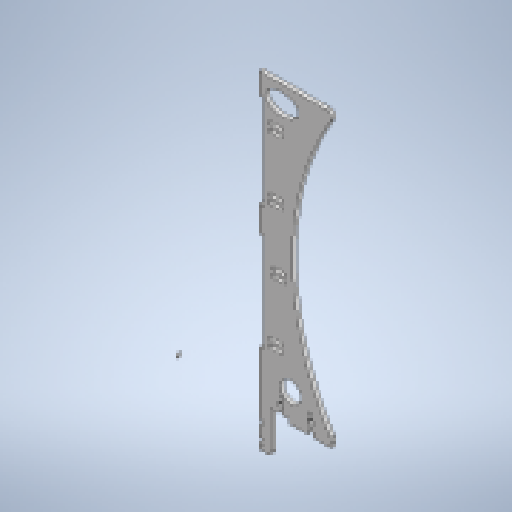
# Autodesk Inventor part: ребро
Saved by Autodesk Inventor 2023.1 (Build 271208000, 208)
## iProperties
Created: 2025-01-17
Part Number: ребро
Material: Типовые
Document SubType Name: Modeling
Designer: Коноваленко
Density: 1 g/cm^3
Appearance: По умолчанию
Author: Коноваленко
Autodesk Inventor part; units mm, degrees
ref_plane "YZ Plane" through (0, 0, 0) normal (1, 0, 0) x (0, 1, 0)
ref_plane "XZ Plane" through (0, 0, 0) normal (0, 1, 0) x (-1, 0, 0)
ref_plane "XY Plane" through (0, 0, 0) normal (0, 0, 1) x (1, 0, 0)
sketch "Эскиз1" plane through (0, 0, 0) normal (0, 0, 1) x (1, 0, 0)
  line L0 (81.8324, 0) -> (81.8324, -4) construction
  line L1 (72.759, -4) -> (11.9953, -4)
  line L2 (11.9953, -4) -> (11.9953, 0) construction
  line L3 (11.9953, 0) -> (81.8324, 0) construction
  line L4 (-75.5314, 0) -> (7.9958, 0) construction
  line L5 (7.9958, 0) -> (7.9958, -4) construction
  line L6 (7.9958, -4) -> (-66.4579, -4)
  line L7 (-75.5314, -4) -> (-75.5314, 0) construction
  line L8 (7.9953, 276) -> (11.9953, 276) construction
  line L9 (-75.5314, 0) -> (81.8324, 0)
  line L10 (72.759, 276) -> (-66.4579, 276)
  arc A0 (-70.7311, 3.5962) -> (-70.7311, 268.4038) centre (-288.6628, 136) ccw
  line L11 (3.1505, 276) -> (3.1505, 0) construction
  arc A1 (77.0322, 268.4038) -> (77.0322, 3.5962) centre (294.9639, 136) ccw
  arc A2 (-66.4579, 276) -> (-70.7311, 268.4038) centre (-66.4579, 271) ccw
  arc A3 (77.0322, 268.4038) -> (72.759, 276) centre (72.759, 271) ccw
  arc A4 (-70.7311, 3.5962) -> (-66.4579, -4) centre (-66.4579, 1) ccw
  arc A5 (72.759, -4) -> (77.0322, 3.5962) centre (72.759, 1) ccw
  point P0 (81.8324, 276)
  point P1 (-75.5314, 276)
  point P2 (-71.3569, 0)
  point P3 (77.658, 0)
  dimension "d0" = 255
  dimension "d1" = 5
  constraints: 24 end point, 16 point on circle, 8 tangent, 6 centre point, 4 point on line, 3 equal radius, 2 midpoint, 1 horizontal, 1 parallel, 1 symmetric about line, 1 other
  measures "d0" radius of A0
  measures "d1" radius of A2
extrude "Выдавливание1" add sketch "Эскиз1" along normal blind 4
sketch "Эскиз2" plane through (0, 0, 4) normal (0, 0, 1) x (1, 0, 0)
  line L0 (-29.8867, 53.1563) -> (-17.8867, 53.1563)
  line L1 (42.1133, 53.1563) -> (42.1133, 54.9927) construction
  line L2 (-29.8867, 50.1563) -> (-29.8867, 53.1563)
  line L3 (6.1133, 50.1563) -> (6.1133, 53.1563)
  line L4 (6.1133, 50.1563) -> (6.1133, 53.1563) construction
  line L5 (-17.8867, 50.1563) -> (-17.8867, 53.1563)
  line L6 (-5.8867, 50.1563) -> (-5.8867, 53.1563)
  line L7 (18.1133, 50.1563) -> (18.1133, 53.1563)
  line L8 (30.1133, 50.1563) -> (30.1133, 53.1563)
  line L9 (-17.8867, 50.1563) -> (-29.8867, 50.1563)
  line L10 (-17.8867, 53.1563) -> (-5.8867, 53.1563) construction
  line L11 (-5.8867, 53.1563) -> (6.1133, 53.1563)
  line L12 (-5.8867, 50.1563) -> (-17.8867, 50.1563) construction
  line L13 (6.1133, 53.1563) -> (18.1133, 53.1563) construction
  line L14 (18.1133, 50.1563) -> (6.1133, 50.1563) construction
  line L15 (18.1133, 53.1563) -> (30.1133, 53.1563)
  line L16 (30.1133, 53.1563) -> (42.1133, 53.1563) construction
  line L17 (30.1133, 50.1563) -> (18.1133, 50.1563)
  line L18 (6.1133, 50.1563) -> (-5.8867, 50.1563)
  line L19 (6.1133, 6.0367) -> (6.1133, 56.3563) construction
  line L20 (-29.8867, 59.3563) -> (-17.8867, 59.3563)
  line L21 (42.1133, 59.3563) -> (42.1133, 56.3563) construction
  line L22 (42.1133, 56.3563) -> (30.1133, 56.3563) construction
  line L23 (-29.8867, 56.3563) -> (-29.8867, 59.3563)
  line L24 (6.1133, 56.3563) -> (6.1133, 59.3563)
  line L25 (6.1133, 56.3563) -> (6.1133, 59.3563) construction
  line L26 (-17.8867, 56.3563) -> (-17.8867, 59.3563)
  line L27 (-5.8867, 56.3563) -> (-5.8867, 59.3563)
  line L28 (18.1133, 56.3563) -> (18.1133, 59.3563)
  line L29 (30.1133, 56.3563) -> (30.1133, 59.3563)
  line L30 (-17.8867, 56.3563) -> (-29.8867, 56.3563)
  line L31 (-17.8867, 59.3563) -> (-5.8867, 59.3563) construction
  line L32 (-5.8867, 59.3563) -> (6.1133, 59.3563)
  line L33 (-5.8867, 56.3563) -> (-17.8867, 56.3563) construction
  line L34 (6.1133, 59.3563) -> (18.1133, 59.3563) construction
  line L35 (18.1133, 56.3563) -> (6.1133, 56.3563) construction
  line L36 (18.1133, 59.3563) -> (30.1133, 59.3563)
  line L37 (30.1133, 59.3563) -> (42.1133, 59.3563) construction
  line L38 (30.1133, 56.3563) -> (18.1133, 56.3563)
  line L39 (6.1133, 56.3563) -> (-5.8867, 56.3563)
  line L40 (6.1133, -16.2034) -> (6.1133, 259.7966) construction
  line L41 (72.759, 276) -> (-66.4579, 276) projected
  line L42 (9.151, 110.1563) -> (9.151, 113.1563)
  line L43 (9.151, 110.1563) -> (9.151, 113.1563) construction
  line L44 (-2.8491, 113.1563) -> (9.151, 113.1563)
  line L45 (9.151, 110.1563) -> (-2.8491, 110.1563)
  line L46 (-2.8491, 110.1563) -> (-2.8491, 113.1563)
  line L47 (-14.8491, 110.1563) -> (-14.8491, 113.1563)
  line L48 (-14.8491, 113.1563) -> (-2.8491, 113.1563) construction
  line L49 (-2.8491, 110.1563) -> (-14.8491, 110.1563) construction
  line L50 (9.151, 55.0001) -> (9.151, 110.1563) construction
  line L51 (21.151, 110.1563) -> (9.151, 110.1563) construction
  line L52 (9.151, 113.1563) -> (21.151, 113.1563) construction
  line L53 (21.151, 110.1563) -> (21.151, 113.1563)
  line L54 (33.151, 110.1563) -> (21.151, 110.1563)
  line L55 (21.151, 113.1563) -> (33.151, 113.1563)
  line L56 (33.151, 110.1563) -> (33.151, 113.1563)
  line L57 (45.1508, 113.1563) -> (45.1508, 110.1563) construction
  line L58 (33.151, 113.1563) -> (45.1508, 113.1563) construction
  line L59 (-26.8491, 113.1563) -> (-14.8491, 113.1563)
  line L60 (-26.8491, 110.1563) -> (-26.8491, 113.1563)
  line L61 (-14.8491, 110.1563) -> (-26.8491, 110.1563)
  line L62 (-14.7363, 116.3563) -> (-14.7363, 119.3563)
  line L63 (-26.7363, 119.3563) -> (-14.7363, 119.3563)
  line L64 (-14.7363, 116.3563) -> (-26.7363, 116.3563)
  line L65 (21.2639, 116.3563) -> (21.2639, 119.3563)
  line L66 (21.2639, 119.3563) -> (33.2639, 119.3563)
  line L67 (33.2639, 116.3563) -> (33.2639, 119.3563)
  line L68 (33.2639, 116.3563) -> (21.2639, 116.3563)
  line L69 (45.2637, 119.3563) -> (45.2637, 116.3563) construction
  line L70 (21.2639, 116.3563) -> (9.2639, 116.3563) construction
  line L71 (9.2639, 119.3563) -> (21.2639, 119.3563) construction
  line L72 (9.2639, 116.3563) -> (9.2639, 119.3563)
  line L73 (9.2639, 116.3563) -> (9.2639, 119.3563) construction
  line L74 (-26.7363, 116.3563) -> (-26.7363, 119.3563)
  line L75 (33.2639, 119.3563) -> (45.2637, 119.3563) construction
  line L76 (-14.7363, 119.3563) -> (-2.7363, 119.3563) construction
  line L77 (-2.7363, 116.3563) -> (-2.7363, 119.3563)
  line L78 (-2.7363, 119.3563) -> (9.2639, 119.3563)
  line L79 (9.2639, 116.3563) -> (-2.7363, 116.3563)
  line L80 (-2.7363, 116.3563) -> (-14.7363, 116.3563) construction
  line L81 (45.2637, 116.3563) -> (33.2639, 116.3563) construction
  line L82 (6.1133, 170.1563) -> (6.1133, 173.1563)
  line L83 (6.1133, 170.1563) -> (6.1133, 173.1563) construction
  line L84 (-5.8867, 173.1563) -> (6.1133, 173.1563)
  line L85 (6.1133, 170.1563) -> (-5.8867, 170.1563)
  line L86 (-5.8867, 170.1563) -> (-5.8867, 173.1563)
  line L87 (-17.8867, 170.1563) -> (-17.8867, 173.1563)
  line L88 (-17.8867, 173.1563) -> (-5.8867, 173.1563) construction
  line L89 (-5.8867, 170.1563) -> (-17.8867, 170.1563) construction
  line L90 (18.1133, 170.1563) -> (6.1133, 170.1563) construction
  line L91 (6.1133, 173.1563) -> (18.1133, 173.1563) construction
  line L92 (18.1133, 170.1563) -> (18.1133, 173.1563)
  line L93 (30.1133, 170.1563) -> (18.1133, 170.1563)
  line L94 (18.1133, 173.1563) -> (30.1133, 173.1563)
  line L95 (30.1133, 170.1563) -> (30.1133, 173.1563)
  line L96 (42.1133, 170.1563) -> (30.1133, 170.1563) construction
  line L97 (42.1133, 173.1563) -> (42.1133, 170.1563) construction
  line L98 (30.1133, 173.1563) -> (42.1133, 173.1563) construction
  line L99 (-29.8867, 173.1563) -> (-17.8867, 173.1563)
  line L100 (-29.8867, 170.1563) -> (-29.8867, 173.1563)
  line L101 (-17.8867, 170.1563) -> (-29.8867, 170.1563)
  line L102 (6.1133, 179.3563) -> (18.1133, 179.3563) construction
  line L103 (18.1133, 176.3563) -> (6.1133, 176.3563) construction
  line L104 (18.1133, 176.3563) -> (18.1133, 179.3563)
  line L105 (30.1133, 176.3563) -> (18.1133, 176.3563)
  line L106 (18.1133, 179.3563) -> (30.1133, 179.3563)
  line L107 (-29.8867, 179.3563) -> (-17.8867, 179.3563)
  line L108 (-17.8867, 176.3563) -> (-29.8867, 176.3563)
  line L109 (-29.8867, 176.3563) -> (-29.8867, 179.3563)
  line L110 (-17.8867, 176.3563) -> (-17.8867, 179.3563)
  line L111 (30.1133, 176.3563) -> (30.1133, 179.3563)
  line L112 (42.1133, 176.3563) -> (30.1133, 176.3563) construction
  line L113 (42.1133, 179.3563) -> (42.1133, 176.3563) construction
  line L114 (30.1133, 179.3563) -> (42.1133, 179.3563) construction
  line L115 (-5.8867, 176.3563) -> (-17.8867, 176.3563) construction
  line L116 (-17.8867, 179.3563) -> (-5.8867, 179.3563) construction
  line L117 (-5.8867, 176.3563) -> (-5.8867, 179.3563)
  line L118 (6.1133, 176.3563) -> (-5.8867, 176.3563)
  line L119 (-5.8867, 179.3563) -> (6.1133, 179.3563)
  line L120 (6.1133, 176.3563) -> (6.1133, 179.3563)
  line L121 (6.1133, 176.3563) -> (6.1133, 179.3563) construction
  line L122 (6.1133, 233.1563) -> (18.1133, 233.1563) construction
  line L123 (18.1133, 230.1563) -> (6.1133, 230.1563) construction
  line L124 (18.1133, 230.1563) -> (18.1133, 233.1563)
  line L125 (30.1133, 230.1563) -> (18.1133, 230.1563)
  line L126 (18.1133, 233.1563) -> (30.1133, 233.1563)
  line L127 (-29.8867, 233.1563) -> (-17.8867, 233.1563)
  line L128 (-17.8867, 230.1563) -> (-29.8867, 230.1563)
  line L129 (-29.8867, 230.1563) -> (-29.8867, 233.1563)
  line L130 (-17.8867, 230.1563) -> (-17.8867, 233.1563)
  line L131 (30.1133, 230.1563) -> (30.1133, 233.1563)
  line L132 (42.1133, 230.1563) -> (30.1133, 230.1563) construction
  line L133 (42.1133, 233.1563) -> (42.1133, 230.1563) construction
  line L134 (30.1133, 233.1563) -> (42.1133, 233.1563) construction
  line L135 (-5.8867, 230.1563) -> (-17.8867, 230.1563) construction
  line L136 (-17.8867, 233.1563) -> (-5.8867, 233.1563) construction
  line L137 (-5.8867, 230.1563) -> (-5.8867, 233.1563)
  line L138 (6.1133, 230.1563) -> (-5.8867, 230.1563)
  line L139 (-5.8867, 233.1563) -> (6.1133, 233.1563)
  line L140 (6.1133, 230.1563) -> (6.1133, 233.1563)
  line L141 (6.1133, 230.1563) -> (6.1133, 233.1563) construction
  line L142 (18.1133, 236.3563) -> (18.1133, 239.3563)
  line L143 (30.1133, 236.3563) -> (18.1133, 236.3563)
  line L144 (18.1133, 239.3563) -> (30.1133, 239.3563)
  line L145 (30.1133, 236.3563) -> (30.1133, 239.3563)
  line L146 (42.1133, 236.3563) -> (30.1133, 236.3563) construction
  line L147 (30.1133, 239.3563) -> (42.1133, 239.3563) construction
  line L148 (42.1133, 239.3563) -> (42.1133, 236.3563) construction
  line L149 (18.1133, 236.3563) -> (6.1133, 236.3563) construction
  line L150 (6.1133, 239.3563) -> (18.1133, 239.3563) construction
  line L151 (6.1133, 236.3563) -> (6.1133, 239.3563)
  line L152 (6.1133, 236.3563) -> (6.1133, 239.3563) construction
  line L153 (6.1133, 236.3563) -> (-5.8867, 236.3563)
  line L154 (-5.8867, 239.3563) -> (6.1133, 239.3563)
  line L155 (-5.8867, 236.3563) -> (-5.8867, 239.3563)
  line L156 (-5.8867, 236.3563) -> (-17.8867, 236.3563) construction
  line L157 (-17.8867, 239.3563) -> (-5.8867, 239.3563) construction
  line L158 (-17.8867, 236.3563) -> (-17.8867, 239.3563)
  line L159 (-29.8867, 239.3563) -> (-17.8867, 239.3563)
  line L160 (-29.8867, 236.3563) -> (-29.8867, 239.3563)
  line L161 (-17.8867, 236.3563) -> (-29.8867, 236.3563)
  arc A0 (-70.7311, 3.5962) -> (-70.7311, 268.4038) centre (-288.6628, 136) ccw construction
  arc A1 (77.0322, 268.4038) -> (77.0322, 3.5962) centre (294.9639, 136) ccw construction
  line L162 (11.994, 110.1563) -> (7.994, 110.1563)
  line L163 (11.9939, 170.1563) -> (7.9939, 170.1563)
  line L164 (11.9939, 230.1563) -> (7.9939, 230.1563)
  point P0 (0, 0)
  point P1 (-29.8867, 51.6563)
  point P2 (-17.8867, 51.6563)
  point P3 (-5.8867, 51.6563)
  point P4 (6.1133, 51.6563)
  point P5 (18.1133, 51.6563)
  point P6 (30.1133, 51.6563)
  point P7 (6.1133, 57.8563)
  point P8 (-29.8867, 57.8563)
  point P9 (-17.8867, 57.8563)
  point P10 (-5.8867, 57.8563)
  point P11 (6.1133, 57.8563)
  point P12 (18.1133, 57.8563)
  point P13 (30.1133, 57.8563)
  point P14 (6.1133, 117.4846)
  point P15 (9.2638, 118.9846)
  point P16 (9.151, 111.6563)
  point P17 (-2.8491, 111.6563)
  point P18 (21.151, 111.6563)
  point P19 (33.151, 111.6563)
  point P20 (-14.8491, 111.6563)
  point P21 (-26.8491, 111.6563)
  point P22 (6.1133, 123.6846)
  point P23 (6.1133, 123.6846)
  point P24 (21.2639, 117.8563)
  point P25 (33.2639, 117.8563)
  point P26 (9.2639, 117.8563)
  point P27 (-26.7363, 117.8563)
  point P28 (-2.7363, 117.8563)
  point P29 (-14.7363, 117.8563)
  point P30 (9.2638, 125.1846)
  point P31 (3.2638, 119.3563)
  point P32 (30.1133, 171.6563)
  point P33 (-17.8867, 171.6563)
  point P34 (-29.8867, 171.6563)
  point P35 (6.1133, 177.1846)
  point P36 (-17.8867, 177.8563)
  point P37 (-29.8867, 177.8563)
  point P38 (30.1133, 177.8563)
  point P39 (6.1133, 177.8563)
  point P40 (6.1133, 225.9846)
  point P41 (6.1133, 225.9846)
  point P42 (18.1133, 231.6563)
  point P43 (-17.8867, 231.6563)
  point P44 (-29.8867, 231.6563)
  point P45 (30.1133, 231.6563)
  point P46 (-5.8867, 231.6563)
  point P47 (18.1133, 237.8563)
  point P48 (30.1133, 237.8563)
  point P49 (-5.8867, 237.8563)
  point P50 (-17.8867, 237.8563)
  point P51 (-29.8867, 237.8563)
  point P52 (6.1133, 232.1846)
  point P53 (6.1133, 225.1563)
  point P54 (0.1133, 179.3563)
  point P55 (9.994, 50.1563)
  point P56 (9.994, 110.1563)
  point P57 (9.9939, 170.1563)
  point P58 (9.9939, 230.1563)
  dimension "d18" = 12
  dimension "d19" = 12
  dimension "d20" = 12
  dimension "d21" = 12
  dimension "d22" = 4.7
  dimension "d23" = 72
  dimension "d25" = 12
  dimension "d26" = 12
  dimension "d27" = 12
  dimension "d28" = 12
  dimension "d39" = 12
  dimension "d40" = 12
  dimension "d41" = 12
  dimension "d42" = 12
  dimension "d44" = 72
  dimension "d46" = 12
  dimension "d47" = 12
  dimension "d48" = 12
  dimension "d49" = 12
  dimension "d54" = 12
  dimension "d59" = 72
  dimension "d60" = 3
  dimension "d61" = 12
  dimension "d66" = 72
  dimension "d68" = 12
  dimension "d69" = 12
  dimension "d71" = 12
  dimension "d74" = 3
  dimension "d75" = 12
  dimension "d76" = 12
  dimension "d78" = 12
  dimension "d79" = 45.8
  dimension "d97" = 3.2
  dimension "d98" = 3
  dimension "d99" = 3.2
  dimension "d100" = 3
  dimension "d101" = 3.2
  dimension "d102" = 3.2
  constraints: 328 end point, 284 parallel, 238 perpendicular, 91 point on line, 48 horizontal, 46 midpoint, 11 vertical, 8 equal length
  measures "d18" distance of point (-29.887, 51.656) point (-17.887, 51.656)
  measures "d19" distance of point (-5.887, 51.656) point (-17.887, 51.656)
  measures "d20" distance of point (6.113, 51.656) point (18.113, 51.656)
  measures "d21" distance of point (30.113, 51.656) point (18.113, 51.656)
  measures "d22" distance from line of point (6.113, 57.856) L11
  measures "d23" distance of L22.start L23.start
  measures "d25" distance of point (-29.887, 57.856) point (-17.887, 57.856)
  measures "d26" distance of point (-5.887, 57.856) point (-17.887, 57.856)
  measures "d27" distance of point (6.113, 57.856) point (18.113, 57.856)
  measures "d28" distance of point (30.113, 57.856) point (18.113, 57.856)
  measures "d39" distance of point (-26.849, 111.656) point (-14.849, 111.656)
  measures "d40" distance of point (-2.849, 111.656) point (-14.849, 111.656)
  measures "d41" distance of point (9.151, 111.656) point (21.151, 111.656)
  measures "d42" distance of point (33.151, 111.656) point (21.151, 111.656)
  measures "d44" distance of L81.start L64.end
  measures "d46" distance of point (-26.736, 117.856) point (-14.736, 117.856)
  measures "d47" distance of point (-2.736, 117.856) point (-14.736, 117.856)
  measures "d48" distance of point (9.264, 117.856) point (21.264, 117.856)
  measures "d49" distance of point (33.264, 117.856) point (21.264, 117.856)
  measures "d54" distance of point (-29.887, 171.656) point (-17.887, 171.656)
  measures "d59" distance of L112.start L109.start
  measures "d60" distance of L114.end L112.start
  measures "d61" distance of point (-29.887, 177.856) point (-17.887, 177.856)
  measures "d66" distance of L132.start L128.end
  measures "d68" distance of point (-29.887, 231.656) point (-17.887, 231.656)
  measures "d69" distance of point (-5.887, 231.656) point (-17.887, 231.656)
  measures "d71" distance of point (30.113, 231.656) point (18.113, 231.656)
  measures "d74" distance of L147.end L146.start
  measures "d75" distance of point (-29.887, 237.856) point (-17.887, 237.856)
  measures "d76" distance of point (-5.887, 237.856) point (-17.887, 237.856)
  measures "d78" distance of point (30.113, 237.856) point (18.113, 237.856)
  measures "d79" vertical distance of point (6.113, 225.156) point (0.113, 179.356)
  measures "d97" distance of L0.start L23.start
  measures "d98" distance of L8.start L8.end
  measures "d99" distance between parallel lines of L55 L68
  measures "d100" distance of L61.end L59.start
  measures "d101" distance between parallel lines of L94 L105
  measures "d102" distance between parallel lines of L126 L143
extrude "Выдавливание2" cut sketch "Эскиз2" against normal blind 10
sketch "Эскиз3" plane through (0, 0, 0) normal (0, 0, -1) x (-1, 0, 0)
  line L0 (29.8867, 239.3563) -> (29.8867, 236.3563)
  line L1 (5.8867, 236.3563) -> (5.8867, 239.3563) construction
  line L2 (29.8867, 239.3563) -> (17.8867, 239.3563) construction
  line L3 (5.8867, 239.3563) -> (17.8867, 239.3563) construction
  line L4 (17.8867, 239.3563) -> (17.8867, 287.0573) construction
  line L5 (-72.759, 276) -> (66.4579, 276) construction
  line L6 (-72.759, 276) -> (66.4579, 276) projected
  line L7 (-3.1505, 276) -> (-3.1505, 0) construction
  ellipse E0 centre (14.7363, 209.3563) end of major axis (14.7363, 194.3563) minor radius 10
  ellipse E1 centre (14.7363, 149.3563) end of major axis (14.7363, 134.3563) minor radius 10
  line L8 (26.9628, 119.3563) -> (14.9628, 119.3563) construction
  line L9 (14.9628, 119.3563) -> (26.9628, 119.3563)
  ellipse E2 centre (-30.1133, 259.231) end of major axis (-46.1133, 259.231) minor radius 10
  line L10 (-30.1133, 236.3563) -> (-30.1133, 239.3563) projected
  line L11 (-18.1133, 239.3563) -> (-30.1133, 239.3563) projected
  line L12 (-30.1133, 239.3563) -> (-30.1133, 283.7222) construction
  line L13 (26.7363, 119.3563) -> (14.7363, 119.3563) projected
  line L14 (14.7363, 119.3563) -> (14.7363, 279.8353) construction
  line L15 (14.7363, 119.3563) -> (175.2153, 119.3563) construction
  line L16 (14.7363, 119.3563) -> (14.7363, -15.3407) construction
  ellipse E3 centre (14.7363, 87.8563) end of major axis (14.7363, 72.8563) minor radius 10
  ellipse E4 centre (14.7363, 29.3563) end of major axis (14.7363, 14.3563) minor radius 10
  line L17 (14.7363, 116.3563) -> (14.7363, 119.3563) projected
  point P0 (0, 0)
  point P1 (-33.2639, 119.3563)
  point P2 (-21.2639, 119.3563)
  point P3 (17.8867, 179.3563)
  point P4 (17.8867, 59.3563)
  point P5 (14.7363, 117.8563)
  dimension "d92" = 16
  dimension "d90" = 160.479
  dimension "d91" = 90
  dimension "d93" = 30
  dimension "d94" = 30
  dimension "d95" = 30
  dimension "d96" = 30
  constraints: 20 end point, 5 point on line, 4 centre point, 3 perpendicular, 3 vertical, 2 horizontal, 2 midpoint, 2 symmetric about line, 2 other
  measures "d90" distance of L13.end L14.end
  measures "d91" angle of L15 L14
  measures "d93" vertical distance of L2.end E0.centre
  measures "d94" vertical distance of E1.centre point (17.887, 179.356)
  measures "d95" distance of E3.centre point (14.736, 117.856)
  measures "d96" vertical distance of E4.centre point (17.887, 59.356)
extrude "Выдавливание3" cut sketch "Эскиз3" against normal blind 10
sketch "Эскиз4" plane through (-71.3569, 0, 0) normal (0, -1, 0) x (1, 0, 0)
  line L0 (91.3569, 4) -> (51.3569, 4)
  line L1 (51.3569, 4) -> (51.3569, 0)
  line L2 (51.3569, 0) -> (91.3569, 0)
  line L3 (91.3569, 0) -> (91.3569, 4)
  line L4 (72.8558, 3.5003) -> (72.8557, 3.5003) projected
  point P0 (71.3569, 0)
  point P1 (0, 4)
  point P2 (149.0149, 4)
  dimension "d103" = 40
  dimension "d104" = 4
  constraints: 8 end point, 2 parallel, 1 horizontal, 1 midpoint, 1 perpendicular
  measures "d103" distance of L1.end L2.end
  measures "d104" distance of L0.end L1.end
extrude "Выдавливание4" add sketch "Эскиз4" along normal blind 20
sketch "Эскиз5" plane through (0, 0, 0) normal (0, 0, -1) x (-1, 0, 0)
  line L0 (0, -20) -> (-20, -20)
  line L1 (-20, -20) -> (-20, -40)
  line L2 (-20, -40) -> (0, -40)
  line L3 (0, -40) -> (0, -20)
  line L4 (20, -20) -> (-20, -20) projected
  point P0 (0, 0)
  point P1 (17, -20)
  point P2 (-17, -20)
  point P3 (0, -20)
  dimension "d108" = 20
  dimension "d109" = 20
  constraints: 8 end point, 2 parallel, 1 horizontal, 1 midpoint, 1 perpendicular
  measures "d108" distance of L2.end L1.end
  measures "d109" distance of L0.end L1.end
extrude "Выдавливание5" add sketch "Эскиз5" against normal blind 4
fillet "Сопряжение2" radius 3 3 edges at (20, -40, 2) (0, -40, 2) (0, -20, 2)
fillet "Сопряжение3" radius 3 1 edges at (-20, -20, 2)
sketch "Эскиз6" plane through (0, 0, 0) normal (0, 0, -1) x (-1, 0, 0)
  line L0 (0, -37) -> (0, -23) projected
  line L1 (-20, 0) -> (-20, -37) projected
  line L2 (0, -23) -> (0, -37) projected
  circle A0 centre (-10, -32) radius 2.55
  circle A1 centre (-10, -17) radius 2.55
  line L3 (-10, -17) -> (-10, -32) construction
  line L4 (-17, -40) -> (-3, -40) projected
  line L5 (-10, -32) -> (-20, -32) construction
  line L6 (-10, -32) -> (0, -32) construction
  point P0 (0, 0)
  point P1 (-10, -40)
  dimension "d121" = 5.1
  dimension "d122" = 5.1
  dimension "d123" = 8
  dimension "d124" = 15
  constraints: 6 end point, 3 point on line, 2 centre point, 1 collinear, 1 midpoint, 1 parallel, 1 perpendicular
  measures "d121" diameter of A1
  measures "d122" diameter of A0
  measures "d123" distance of point (-10, -40) L3.end
  measures "d124" distance of L3.start L3.end
extrude "Выдавливание6" cut sketch "Эскиз6" against normal blind 4
sketch "Эскиз7" plane through (0, 0, 0) normal (0, 0, -1) x (-1, 0, 0)
  circle A0 centre (-38.6107, 23.1063) radius 10
  point P0 (0, 0)
  dimension "d125" = 20
  constraints: 1 centre point
  measures "d125" diameter of A0
extrude "Выдавливание7" cut sketch "Эскиз7" against normal blind 4
sketch "Эскиз8" plane through (77.658, 0, 0) normal (0, -1, 0) x (1, 0, 0)
  line L0 (-57.658, 4) -> (0, 4) construction
  line L1 (-57.658, 0) -> (0, 0) construction
  line L2 (0, 4) -> (-17.5, 4)
  line L3 (-17.5, 4) -> (-17.5, 0)
  line L4 (-17.5, 0) -> (0, 0)
  line L5 (0, 0) -> (0, 4)
  line L6 (-22.5, 4) -> (-40, 4)
  line L7 (-40, 4) -> (-40, 0)
  line L8 (-40, 0) -> (-22.5, 0)
  line L9 (-22.5, 0) -> (-22.5, 4)
  line L10 (-148.3891, 0) -> (-149.1159, 0) projected
  line L11 (-149.0149, 4) -> (-97.658, 4) projected
  line L12 (-149.1159, 0) -> (-131.6159, 0)
  line L13 (-131.6159, 0) -> (-131.6159, 4)
  line L14 (-131.6159, 4) -> (-149.1159, 4)
  line L15 (-149.1159, 4) -> (-149.1159, 0)
  line L16 (-149.0149, 0) -> (-97.658, 0) projected
  line L17 (-126.6159, 0) -> (-109.1159, 0)
  line L18 (-109.1159, 0) -> (-109.1159, 4)
  line L19 (-109.1159, 4) -> (-126.6159, 4)
  line L20 (-126.6159, 4) -> (-126.6159, 0)
  point P0 (-77.658, 0)
  point P1 (-17.5, 4)
  point P2 (-131.6159, 2)
  point P3 (-126.6159, 2)
  point P4 (-126.6159, 4)
  dimension "d128" = 17.5
  dimension "d137" = 17.5
  dimension "d138" = 5
  dimension "d139" = 17.5
  dimension "d140" = 17.5
  dimension "d141" = 5
  constraints: 32 end point, 8 parallel, 6 point on line, 4 horizontal, 4 perpendicular, 2 midpoint
  measures "d128" distance of L4.end L3.end
  measures "d137" distance of L6.start L6.end
  measures "d138" distance between parallel lines of L9 L3
  measures "d139" distance of L14.end L13.end
  measures "d140" distance of L19.end L18.end
  measures "d141" distance of point (-131.616, 2) point (-126.616, 2)
extrude "Выдавливание8" add sketch "Эскиз8" along normal blind 4 contours L5 L4 L3 L2 | L9 L8 L7 L6 | L10 L15 L14 L11 L13 L12 | L20 L11 L18 L16
sketch "Эскиз9" plane through (0, 0, 4) normal (0, 0, 1) x (1, 0, 0)
  line L0 (-27.304, 0) -> (-24.154, 0)
  line L1 (-24.154, 15) -> (-27.304, 15)
  line L2 (-22.979, 8.8) -> (-22.979, 6.5)
  line L3 (-28.479, 6.5) -> (-28.479, 8.8)
  line L4 (-25.729, 15) -> (-25.729, 0) construction
  line L5 (-28.479, 8.8) -> (-27.304, 8.8)
  line L6 (-24.154, 8.8) -> (-22.979, 8.8)
  line L7 (-27.304, 15) -> (-27.304, 8.8)
  line L8 (-27.304, 6.5) -> (-27.304, 0)
  line L9 (-22.979, 6.5) -> (-24.154, 6.5)
  line L10 (-27.304, 6.5) -> (-28.479, 6.5)
  line L11 (-24.154, 0) -> (-24.154, 6.5)
  line L12 (-24.154, 8.8) -> (-24.154, 15)
  line L13 (-52.8263, 0) -> (-50.0896, 0)
  line L14 (-49.8829, 14.9986) -> (-53.0329, 14.9986)
  line L15 (-48.7079, 8.8) -> (-48.7079, 6.5)
  line L16 (-54.2079, 6.5) -> (-54.2079, 8.8)
  line L17 (-51.4579, 14.9986) -> (-51.4579, 0) construction
  line L18 (-54.2079, 8.8) -> (-53.0329, 8.8)
  line L19 (-49.8829, 8.8) -> (-48.7079, 8.8)
  line L20 (-53.0329, 14.9986) -> (-53.0329, 8.8)
  line L21 (-52.8263, 6.5) -> (-52.8263, 0)
  line L22 (-48.7079, 6.5) -> (-50.0896, 6.5)
  line L23 (-52.8263, 6.5) -> (-54.2079, 6.5)
  line L24 (-50.0896, 0) -> (-50.0896, 6.5)
  line L25 (-49.8829, 8.8) -> (-49.8829, 14.9986)
  line L26 (-53.9579, 0) -> (-48.9579, 0) projected
  line L27 (-52.8263, 6.5) -> (-50.0896, 6.5) construction
  line L28 (30.404, 0) -> (27.254, 0)
  line L29 (27.254, 15) -> (30.404, 15)
  line L30 (20, 0) -> (37.658, 0) projected
  line L31 (26.079, 6.5) -> (26.079, 8.8)
  line L32 (31.579, 8.8) -> (31.579, 6.5)
  line L33 (28.829, 15) -> (28.829, 0) construction
  line L34 (26.079, 8.8) -> (27.254, 8.8)
  line L35 (30.404, 8.8) -> (31.579, 8.8)
  line L36 (27.254, 0) -> (27.254, 6.5)
  line L37 (27.254, 8.8) -> (27.254, 15)
  line L38 (30.404, 15) -> (30.404, 8.8)
  line L39 (30.404, 6.5) -> (30.404, 0)
  line L40 (31.579, 6.5) -> (30.404, 6.5)
  line L41 (27.254, 6.5) -> (26.079, 6.5)
  line L42 (59.233, 0) -> (56.083, 0)
  line L43 (56.083, 15) -> (59.233, 15)
  line L44 (60.408, 6.5) -> (60.408, 8.8)
  line L45 (54.908, 8.8) -> (54.908, 6.5)
  line L46 (55.158, 0) -> (60.158, 0) projected
  line L47 (57.658, 15) -> (57.658, 0) construction
  line L48 (60.408, 8.8) -> (59.233, 8.8)
  line L49 (56.083, 8.8) -> (54.908, 8.8)
  line L50 (56.083, 0) -> (56.083, 6.5)
  line L51 (56.083, 8.8) -> (56.083, 15)
  line L52 (54.908, 6.5) -> (56.083, 6.5)
  line L53 (59.233, 6.5) -> (60.408, 6.5)
  line L54 (59.233, 15) -> (59.233, 8.8)
  line L55 (59.233, 6.5) -> (59.233, 0)
  point P0 (0, 0)
  point P1 (-31.4579, 0)
  point P2 (-49.3988, 6.5)
  dimension "d132" = 15
  dimension "d133" = 3.15
  dimension "d134" = 2.3
  dimension "d135" = 5.5
  dimension "d142" = 15
  dimension "d143" = 3.15
  dimension "d144" = 2.3
  dimension "d145" = 5.5
  dimension "d146" = 6.5
  dimension "d154" = 3.15
  dimension "d155" = 15
  dimension "d156" = 5.5
  dimension "d157" = 2.3
  dimension "d159" = 3.15
  dimension "d160" = 15
  dimension "d161" = 5.5
  dimension "d162" = 2.3
  constraints: 106 end point, 40 parallel, 16 perpendicular, 13 horizontal, 12 midpoint, 5 equal length, 4 vertical
  measures "d132" distance of L0.end L1.start
  measures "d133" distance of L1.start L1.end
  measures "d134" distance of L2.start L2.end
  measures "d135" distance of L3.end L2.start
  measures "d142" distance of L24.start L25.end
  measures "d143" distance of L25.end L14.end
  measures "d144" distance of L15.start L15.end
  measures "d145" distance of L16.end L15.start
  measures "d146" vertical distance of L24.start point (-49.399, 6.5)
  measures "d154" distance of L29.start L29.end
  measures "d155" distance of L28.end L29.start
  measures "d156" distance of L31.end L32.start
  measures "d157" distance of L31.start L31.end
  measures "d159" distance of L43.start L43.end
  measures "d160" distance of L42.end L43.start
  measures "d161" distance of L45.start L44.end
  measures "d162" distance of L44.end L44.start
extrude "Выдавливание9" cut sketch "Эскиз9" against normal blind 4
sketch "Эскиз11" plane through (0, 0, 4) normal (0, 0, 1) x (1, 0, 0)
  line L0 (12.0209, 165.1563) -> (8.0209, 165.1563) construction
  line L1 (8.021, 0) -> (8.021, 45.1563)
  ellipse E0 centre (-14.7363, 149.3563) end of major axis (-14.7363, 134.3563) minor radius 10 construction
  ellipse E1 centre (-14.7363, 87.8563) end of major axis (-14.7363, 72.8563) minor radius 10 construction
  ellipse E2 centre (-14.7363, 209.3563) end of major axis (-14.7363, 194.3563) minor radius 10 construction
  line L2 (6.1133, 236.3563) -> (6.1133, 239.3563) construction
  line L3 (6.1133, 239.3563) -> (-5.8867, 239.3563) construction
  line L4 (-5.8867, 239.3563) -> (-5.8867, 236.3563) construction
  line L5 (-5.8867, 236.3563) -> (6.1133, 236.3563) construction
  line L6 (-2.8491, 110.1563) -> (9.151, 110.1563) construction
  line L7 (9.151, 110.1563) -> (9.151, 113.1563) construction
  line L8 (9.151, 113.1563) -> (-2.8491, 113.1563) construction
  line L9 (-2.8491, 113.1563) -> (-2.8491, 110.1563) construction
  line L10 (-29.8867, 176.3563) -> (-17.8867, 176.3563) construction
  line L11 (-17.8867, 176.3563) -> (-17.8867, 179.3563) construction
  line L12 (-17.8867, 179.3563) -> (-29.8867, 179.3563) construction
  line L13 (-29.8867, 179.3563) -> (-29.8867, 176.3563) construction
  line L14 (-26.7363, 116.3563) -> (-14.7363, 116.3563) construction
  line L15 (-14.7363, 116.3563) -> (-14.7363, 119.3563) construction
  line L16 (-14.7363, 119.3563) -> (-26.7363, 119.3563) construction
  line L17 (-26.7363, 119.3563) -> (-26.7363, 116.3563) construction
  line L18 (-29.8867, 56.3563) -> (-17.8867, 56.3563) construction
  line L19 (-17.8867, 56.3563) -> (-17.8867, 59.3563) construction
  line L20 (-17.8867, 59.3563) -> (-29.8867, 59.3563) construction
  line L21 (-29.8867, 59.3563) -> (-29.8867, 56.3563) construction
  line L22 (-17.8867, 53.1563) -> (-29.8867, 53.1563) construction
  line L23 (30.1133, 50.1563) -> (30.1133, 53.1563) construction
  line L24 (30.1133, 53.1563) -> (18.1133, 53.1563) construction
  line L25 (18.1133, 53.1563) -> (18.1133, 50.1563) construction
  line L26 (18.1133, 50.1563) -> (30.1133, 50.1563) construction
  line L27 (-5.8867, 176.3563) -> (6.1133, 176.3563) construction
  line L28 (6.1133, 176.3563) -> (6.1133, 179.3563) construction
  line L29 (6.1133, 179.3563) -> (-5.8867, 179.3563) construction
  line L30 (-5.8867, 179.3563) -> (-5.8867, 176.3563) construction
  line L31 (-26.8491, 110.1563) -> (-14.8491, 110.1563) construction
  line L32 (-14.8491, 110.1563) -> (-14.8491, 113.1563) construction
  line L33 (-14.8491, 113.1563) -> (-26.8491, 113.1563) construction
  line L34 (-26.8491, 113.1563) -> (-26.8491, 110.1563) construction
  line L35 (30.1133, 176.3563) -> (30.1133, 179.3563) construction
  line L36 (30.1133, 179.3563) -> (18.1133, 179.3563) construction
  line L37 (18.1133, 179.3563) -> (18.1133, 176.3563) construction
  line L38 (18.1133, 176.3563) -> (30.1133, 176.3563) construction
  line L39 (-29.8867, 236.3563) -> (-17.8867, 236.3563) construction
  line L40 (-17.8867, 236.3563) -> (-17.8867, 239.3563) construction
  line L41 (-17.8867, 239.3563) -> (-29.8867, 239.3563) construction
  line L42 (-29.8867, 239.3563) -> (-29.8867, 236.3563) construction
  line L43 (6.1133, 230.1563) -> (6.1133, 233.1563) construction
  line L44 (6.1133, 233.1563) -> (-5.8867, 233.1563) construction
  line L45 (-5.8867, 233.1563) -> (-5.8867, 230.1563) construction
  line L46 (-5.8867, 230.1563) -> (6.1133, 230.1563) construction
  line L47 (6.1133, 170.1563) -> (6.1133, 173.1563) construction
  line L48 (6.1133, 173.1563) -> (-5.8867, 173.1563) construction
  line L49 (-5.8867, 173.1563) -> (-5.8867, 170.1563) construction
  line L50 (-5.8867, 170.1563) -> (6.1133, 170.1563) construction
  line L51 (21.2639, 119.3563) -> (21.2639, 116.3563) construction
  line L52 (30.1133, 170.1563) -> (30.1133, 173.1563) construction
  line L53 (30.1133, 173.1563) -> (18.1133, 173.1563) construction
  line L54 (18.1133, 173.1563) -> (18.1133, 170.1563) construction
  line L55 (18.1133, 170.1563) -> (30.1133, 170.1563) construction
  line L56 (-5.8867, 56.3563) -> (6.1133, 56.3563) construction
  line L57 (6.1133, 56.3563) -> (6.1133, 59.3563) construction
  line L58 (6.1133, 59.3563) -> (-5.8867, 59.3563) construction
  line L59 (-5.8867, 59.3563) -> (-5.8867, 56.3563) construction
  line L60 (-5.8867, 50.1563) -> (6.1133, 50.1563) construction
  line L61 (6.1133, 50.1563) -> (6.1133, 53.1563) construction
  line L62 (6.1133, 53.1563) -> (-5.8867, 53.1563) construction
  line L63 (-5.8867, 53.1563) -> (-5.8867, 50.1563) construction
  line L64 (30.1133, 56.3563) -> (30.1133, 59.3563) construction
  line L65 (30.1133, 59.3563) -> (18.1133, 59.3563) construction
  line L66 (18.1133, 59.3563) -> (18.1133, 56.3563) construction
  line L67 (18.1133, 56.3563) -> (30.1133, 56.3563) construction
  line L68 (-17.8867, 170.1563) -> (-17.8867, 173.1563) construction
  line L69 (-17.8867, 173.1563) -> (-29.8867, 173.1563) construction
  line L70 (-29.8867, 173.1563) -> (-29.8867, 170.1563) construction
  line L71 (-29.8867, 170.1563) -> (-17.8867, 170.1563) construction
  line L72 (-2.7363, 116.3563) -> (9.2639, 116.3563) construction
  line L73 (9.2639, 116.3563) -> (9.2639, 119.3563) construction
  line L74 (9.2639, 119.3563) -> (-2.7363, 119.3563) construction
  line L75 (-2.7363, 119.3563) -> (-2.7363, 116.3563) construction
  line L76 (21.151, 113.1563) -> (21.151, 110.1563) construction
  line L77 (-17.8867, 230.1563) -> (-17.8867, 233.1563) construction
  line L78 (-17.8867, 233.1563) -> (-29.8867, 233.1563) construction
  line L79 (-29.8867, 233.1563) -> (-29.8867, 230.1563) construction
  line L80 (-29.8867, 230.1563) -> (-17.8867, 230.1563) construction
  line L81 (8.0209, 276) -> (8.0209, 256)
  line L82 (12.0209, 256) -> (12.0209, 165.1563)
  line L83 (12.0209, 165.1563) -> (8.0209, 165.1563)
  line L84 (8.0209, 165.1563) -> (8.0209, 140.1563)
  line L85 (8.0209, 140.1563) -> (12.0209, 140.1563)
  line L86 (8.021, 45.1563) -> (8.021, 0) construction
  line L87 (8.0209, 256) -> (12.0209, 256)
  line L88 (12.0209, 45.1563) -> (8.021, 45.1563)
  line L89 (12.0209, 140.1563) -> (12.0209, 45.1563)
  arc A0 (-70.7311, 3.5962) -> (-70.7311, 268.4038) centre (-288.6628, 136) ccw projected
  line L90 (72.759, 276) -> (-66.4579, 276) projected
  arc A1 (-66.4579, 276) -> (-70.7311, 268.4038) centre (-66.4579, 271) ccw projected
  arc A2 (-70.7311, 3.5962) -> (-71.3569, 0) centre (-66.4579, 1) ccw projected
  line L91 (8.021, 0) -> (8.021, -81.5926)
  line L92 (8.021, -81.5926) -> (-71.3569, -81.5926)
  line L93 (-71.3569, -81.5926) -> (-71.3569, 0)
  constraints: 186 end point, 4 perpendicular, 3 horizontal, 3 vertical, 1 collinear, 6 other
extrude "Выдавливание10" cut sketch "Эскиз11" against normal blind 10
